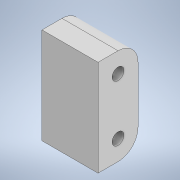
# Autodesk Inventor part: damping_system_housing_connector
Saved by Autodesk Inventor 2021 (Build 250183000, 183)
## iProperties
Created: 2020-10-27
Part Number: damping_system_housing_connector
Material: Generic
Document SubType Name: Modeling
Designer: Mateusz
Density: 1 g/cm^3
Appearance: Default
Author: Mateusz
Autodesk Inventor part; units mm, degrees
ref_plane "YZ Plane" through (0, 0, 0) normal (1, 0, 0) x (0, 1, 0)
ref_plane "XZ Plane" through (0, 0, 0) normal (0, 1, 0) x (-1, 0, 0)
ref_plane "XY Plane" through (0, 0, 0) normal (0, 0, 1) x (1, 0, 0)
sketch "Sketch1" plane through (0, 0, 0) normal (1, 0, 0) x (0, 1, 0)
  line L0 (0, 0) -> (40, 0)
  circle A0 centre (0, 0) radius 4.25
  circle A1 centre (0, 0) radius 11.25
  circle A2 centre (40, 0) radius 4.25
  circle A3 centre (40, 0) radius 11.25
  arc A4 (40, 14.25) -> (54.25, 0) centre (40, 0) ccw
  arc A5 (-14.25, 0) -> (0, 14.25) centre (0, 0) ccw
  line L1 (40, -14.25) -> (0, -14.25)
  line L2 (0, 14.25) -> (40, 14.25)
  line L3 (54.25, 0) -> (54.25, 14.25)
  line L4 (54.25, 14.25) -> (40, 14.25)
  line L5 (-14.25, 0) -> (-14.25, 14.25)
  line L6 (-14.25, 14.25) -> (0, 14.25)
  line L7 (40, -11.25) -> (0, -11.25)
  dimension "d2" = 22.5
  dimension "d4" = 22.5
  dimension "d0" = 40
  dimension "d1" = 8.5
  dimension "d3" = 8.5
  dimension "d5" = 28.5
  dimension "d6" = 28.5
  constraints: 16 end point, 6 coincident, 6 point on circle, 5 tangent, 4 centre point, 4 horizontal, 4 perpendicular, 2 point on line, 2 vertical alignment, 1 parallel, 4 other
  measures "d0" distance of L0.start L0.end
  measures "d1" diameter of A0
  measures "d3" diameter of A2
  measures "d5" diameter of A4
  measures "d6" diameter of A5
extrude "Extrusion1" add sketch "Sketch1" along normal blind 3 contours A1 L7 A5 L5 L6 L0 | L0 A5 L7 A1 | A5 L2 A4 L0 | L0 A4 L7 A5 | A4 L4 L3 L7 A3 L0 | L0 A3 L7 A4 | L7 A4 L1 A5
sketch "Sketch2" plane through (0, -14.25, 14.25) normal (0, 0, 1) x (1, 0, 0)
  line L0 (0, 68.5) -> (0, 0) projected
  line L1 (0, 0) -> (-34, 0)
  line L2 (-34, 0) -> (-34, 68.5)
  line L3 (-34, 68.5) -> (0, 68.5)
  point P0 (0, 14.25)
  dimension "d9" = 34
  constraints: 6 end point, 2 perpendicular, 1 horizontal
  measures "d9" distance of L0.end L1.end
extrude "Extrusion2" add sketch "Sketch2" against normal blind 3
sketch "Sketch3" plane through (-34, -14.25, 14.25) normal (-1, 0, 0) x (0, 0, 1)
  circle A0 centre (-14.25, 54.25) radius 11.25 projected
  circle A1 centre (-14.25, 54.25) radius 11.25
  circle A2 centre (-14.25, 14.25) radius 11.25 projected
  circle A3 centre (-14.25, 14.25) radius 11.25
  circle A4 centre (-14.25, 14.25) radius 14.25
  arc A5 (-14.25, 68.5) -> (-28.5, 54.25) centre (-14.25, 54.25) ccw projected
  circle A6 centre (-14.25, 54.25) radius 14.25
  line L0 (-28.5, 14.25) -> (-28.5, 54.25) projected
  line L1 (-28.5, 54.25) -> (-28.5, 14.25)
  line L2 (0, 0) -> (-14.25, 0) projected
  line L3 (-14.25, 0) -> (0, 0)
  line L4 (0, 68.5) -> (0, 0) projected
  line L5 (0, 0) -> (0, 68.5)
  line L6 (-14.25, 68.5) -> (0, 68.5) projected
  line L7 (0, 68.5) -> (-14.25, 68.5)
  constraints: 8 end point, 4 coincident, 4 collinear, 3 centre point, 2 tangent, 1 horizontal, 1 vertical, 1 vertical alignment, 2 other
extrude "Extrusion3" add sketch "Sketch3" along normal blind 3
extrude "Extrusion4" add sketch "Sketch3" against normal up to surface (34 mm away) contours A0 | A2 | A4 | L4 L2 A4 | A4 L0 A6 L4 | A6 A5 | A6 L6 L4
sketch "Sketch4" plane through (0, 40, 0) normal (1, 0, 0) x (0, 0, -1)
  circle A0 centre (0, 0) radius 4.25
  circle A1 centre (0, -40) radius 4.25
  dimension "d16" = 8.5
  dimension "d17" = 8.5
  constraints: 2 centre point, 1 coincident
  measures "d16" diameter of A0
  measures "d17" diameter of A1
extrude "Extrusion5" cut sketch "Sketch4" against normal up to surface (37 mm away)
sketch "Sketch7" plane through (3, 0, 0) normal (1, 0, 0) x (0, 0, -1)
  line L0 (0, 54.25) -> (-14.25, 54.25) projected
  line L1 (0, 54.25) -> (14.25, 54.25)
  arc A0 (14.25, 40) -> (0, 54.25) centre (0, 40) ccw projected
  line L2 (14.25, 54.25) -> (14.25, 40)
  point P0 (0, 0)
  constraints: 4 end point, 2 tangent, 1 horizontal, 1 perpendicular
extrude "Extrusion8" cut sketch "Sketch7" against normal up to surface (40 mm away)
sketch "Sketch8" plane through (0, 40, 0) normal (1, 0, 0) x (0, 0, -1)
  circle A0 centre (0, 0) radius 4.25 projected
  circle A1 centre (0, 0) radius 11.25 projected
  circle A2 centre (0, -40) radius 4.25 projected
  circle A3 centre (0, -40) radius 11.25 projected
extrude "Extrusion9" add sketch "Sketch8" along normal up to surface (3 mm away)
sketch "Sketch9" plane through (-34, 40, 0) normal (-1, 0, 0) x (0, 0, 1)
  circle A0 centre (0, 0) radius 4.25 projected
  circle A1 centre (0, 0) radius 11.25 projected
  circle A2 centre (0, -40) radius 4.25 projected
  circle A3 centre (0, -40) radius 11.25 projected
extrude "Extrusion10" add sketch "Sketch9" along normal up to surface (3 mm away)
body "Solid1"
